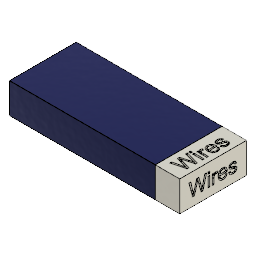
_7.12d72cee-9055-4304-aa3c-481a48856ccf (Autodesk Fusion 360 design; units mm, degrees)
Autodesk Fusion 360 part; units mm, degrees
sketch "Sketch1" plane through (0, 0, 0) normal (0, 0, 1) x (1, 0, 0)
  line L0 (-38.1, 17.4625) -> (38.1, 17.4625)
  line L1 (38.1, 17.4625) -> (38.1, -17.4625)
  line L2 (38.1, -17.4625) -> (-38.1, -17.4625)
  line L3 (-38.1, -17.4625) -> (-38.1, 17.4625)
  line L4 (-38.1, 17.4625) -> (38.1, -17.4625) construction
  line L5 (38.1, 17.4625) -> (-38.1, -17.4625) construction
  line L6 (38.1, 17.4625) -> (50.8, 17.4625)
  line L7 (50.8, 17.4625) -> (50.8, -17.4625)
  line L8 (50.8, -17.4625) -> (38.1, -17.4625)
  dimension "d1" = 76.2
  dimension "d2" = 34.925
  dimension "d3" = 12.7
  constraint horizontal L0
  constraint perpendicular L0 L1
  constraint perpendicular L1 L2
  constraint perpendicular L0 L3
  constraint coincident L3 L2.end
  constraint coincident L2.end L3.start
  constraint coincident origin L5
  constraint coincident origin L4
  constraint perpendicular L1 L6
  constraint perpendicular L6 L7
  constraint horizontal L8
  measures "d1" distance of L0.start L0.end
  measures "d2" distance of L0.start L2.end
  measures "d3" distance of L0.end L6.end
extrude "Extrude1" add sketch "Sketch1" along normal mid plane 15.875 contours L0 L1 L2 L3 makes body 1
extrude "Extrude2" add sketch "Sketch1" along normal mid plane 15.875 separate body contours L1 L6 L7 L8 makes body 2
sketch "Sketch2" plane through (0, 0, 7.9375) normal (0, 0, 1) x (-1, 0, 0)
  line L0 (-38.1, -17.4625) -> (-38.1, 17.4625)
  line L1 (-38.1, 17.4625) -> (-50.8, 17.4625)
  line L2 (-50.8, 17.4625) -> (-50.8, -17.4625)
  line L3 (-50.8, -17.4625) -> (-38.1, -17.4625)
  line L4 (-48.2643, 12.8881) -> (-48.2643, -12.1559) construction
  line L5 (-48.2643, -12.1559) -> (-38.2643, -12.1559) construction
  line L6 (-38.2643, -12.1559) -> (-38.2643, 12.8881) construction
  line L7 (-38.2643, 12.8881) -> (-48.2643, 12.8881) construction
  text T0 "Wires" font "Arial" height 10 align ink ink in box 0 x 0 at (-48.2443, 12.8781) x (0, -1) y (1, 0) spacing 1 height is em
  constraint perpendicular L4 L5
  constraint parallel L4 L6
  constraint parallel L5 L7
extrude "Extrude3" cut sketch "Sketch2" against normal blind 1.27 text T0 bodies 2
sketch "Sketch3" plane through (0, 0, -7.9375) normal (0, 0, -1) x (1, 0, 0)
  line L0 (38.1, 17.4625) -> (38.1, -17.4625)
  line L1 (38.1, -17.4625) -> (50.8, -17.4625)
  line L2 (50.8, -17.4625) -> (50.8, 17.4625)
  line L3 (50.8, 17.4625) -> (38.1, 17.4625)
  line L4 (48.993, -12.4624) -> (48.993, 12.5816) construction
  line L5 (48.993, 12.5816) -> (38.993, 12.5816) construction
  line L6 (38.993, 12.5816) -> (38.993, -12.4624) construction
  line L7 (38.993, -12.4624) -> (48.993, -12.4624) construction
  text T0 "Wires" font "Arial" height 10 align ink ink in box 0 x 0 at (48.973, -12.4524) x (0, 1) y (-1, 0) spacing 1 height is em
  constraint perpendicular L4 L5
  constraint parallel L4 L6
  constraint parallel L5 L7
extrude "Extrude4" cut sketch "Sketch3" against normal blind 1.27 text T0 bodies 2
sketch "Sketch4" plane through (50.8, 0, 0) normal (1, 0, 0) x (0, 1, 0)
  line L0 (17.4625, -7.9375) -> (17.4625, 7.9375)
  line L1 (17.4625, 7.9375) -> (-17.4625, 7.9375)
  line L2 (-17.4625, 7.9375) -> (-17.4625, -7.9375)
  line L3 (-17.4625, -7.9375) -> (17.4625, -7.9375)
  line L4 (-12.652, -3.6746) -> (12.392, -3.6746) construction
  line L5 (12.392, -3.6746) -> (12.392, 6.3254) construction
  line L6 (12.392, 6.3254) -> (-12.652, 6.3254) construction
  line L7 (-12.652, 6.3254) -> (-12.652, -3.6746) construction
  text T0 "Wires" font "Arial" height 10 align ink ink in box 0 x 0 at (-12.642, -3.6546) x (1, 0) y (0, 1) spacing 1 height is em
  constraint perpendicular L4 L5
  constraint parallel L4 L6
  constraint parallel L5 L7
extrude "Extrude5" cut sketch "Sketch4" against normal blind 1.27 text T0 bodies 2
